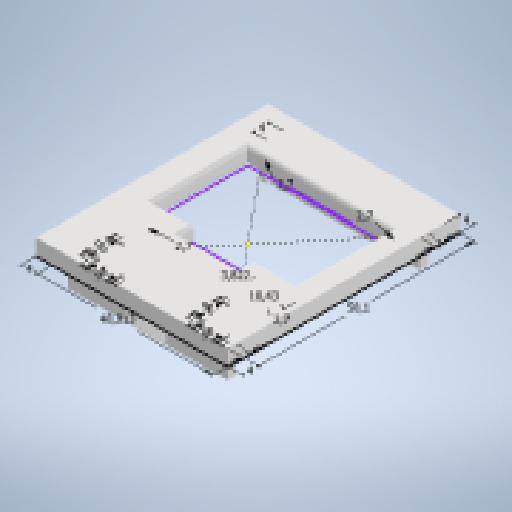
# Autodesk Inventor part: Deckel
Saved by Autodesk Inventor 2024 (Build 280153000, 153)
## iProperties
Created: 2025-05-07
Part Number: Deckel
Material: Generisch
Document SubType Name: Modeling
Designer: tobia
Density: 1 g/cm^3
Appearance: Vorgabe
Author: tobia
Autodesk Inventor part; units mm, degrees
ref_plane "YZ Plane" through (0, 0, 0) normal (1, 0, 0) x (0, 1, 0)
ref_plane "XZ Plane" through (0, 0, 0) normal (0, 1, 0) x (-1, 0, 0)
ref_plane "XY Plane" through (0, 0, 0) normal (0, 0, 1) x (1, 0, 0)
sketch "Skizze1" plane through (0, 0, 0) normal (0, 0, 1) x (1, 0, 0)
  line L0 (-24.0065, 29.05) -> (24.0065, 29.05)
  line L1 (24.0065, 29.05) -> (24.0065, -29.05)
  line L2 (24.0065, -29.05) -> (-24.0065, -29.05)
  line L3 (-24.0065, -29.05) -> (-24.0065, 29.05)
  line L4 (-24.0065, 29.05) -> (24.0065, -29.05) construction
  line L5 (24.0065, 29.05) -> (-24.0065, -29.05) construction
  line L6 (-24.0065, 29.05) -> (-20.0065, 29.05)
  line L7 (-20.0065, 29.05) -> (-20.0065, -29.05)
  line L8 (-20.0065, -29.05) -> (-24.0065, -29.05)
  line L9 (-24.0065, -29.05) -> (-24.0065, 29.05)
  line L10 (-20.0065, -29.05) -> (24.0065, -29.05)
  line L11 (24.0065, -29.05) -> (24.0065, -25.05)
  line L12 (24.0065, -25.05) -> (-20.0065, -25.05)
  line L13 (-20.0065, -25.05) -> (-20.0065, -29.05)
  line L14 (24.0065, -25.05) -> (20.0065, -25.05)
  line L15 (20.0065, -25.05) -> (20.0065, 29.05)
  line L16 (20.0065, 29.05) -> (24.0065, 29.05)
  line L17 (24.0065, 29.05) -> (24.0065, -25.05)
  line L18 (20.0065, 29.05) -> (-20.0065, 29.05)
  line L19 (-20.0065, 29.05) -> (-20.0065, 25.05)
  line L20 (-20.0065, 25.05) -> (20.0065, 25.05)
  line L21 (20.0065, 25.05) -> (20.0065, 29.05)
  line L22 (-20.0065, 25.05) -> (20.0065, 25.05)
  line L23 (20.0065, 25.05) -> (20.0065, 23.05)
  line L24 (20.0065, 23.05) -> (-20.0065, 23.05)
  line L25 (-20.0065, 23.05) -> (-20.0065, 25.05)
  line L26 (-20.0065, -25.05) -> (20.0065, -25.05)
  line L27 (20.0065, -25.05) -> (20.0065, -23.05)
  line L28 (20.0065, -23.05) -> (-20.0065, -23.05)
  line L29 (-20.0065, -23.05) -> (-20.0065, -25.05)
  line L30 (-24.0065, 29.05) -> (24.0065, 29.05)
  line L31 (24.0065, 29.05) -> (24.0065, -29.05)
  line L32 (24.0065, -29.05) -> (-24.0065, -29.05)
  line L33 (-24.0065, -29.05) -> (-24.0065, 29.05)
  circle A0 centre (-14.7085, 19.65) radius 1.35
  circle A1 centre (15.6927, 19.65) radius 1.35
  circle A2 centre (-14.7085, -8.9604) radius 1.35
  circle A3 centre (15.6927, -8.9604) radius 1.35
  line L34 (-17.3399, 17.2285) -> (18.4839, 17.2285)
  line L35 (18.4839, 17.2285) -> (18.4839, -6.4884)
  line L36 (18.4839, -6.4884) -> (-17.3399, -6.4884)
  line L37 (-17.3399, -6.4884) -> (-17.3399, 17.2285)
  line L38 (-17.3399, -6.4884) -> (-6.9094, -6.4884)
  line L39 (-6.9094, -10.3104) -> (-6.9094, -6.4884)
  line L40 (18.4839, -6.4884) -> (8.0539, -6.4884)
  line L41 (8.0539, -6.4884) -> (8.0539, -10.3104)
  line L42 (8.0539, -10.3104) -> (-6.9094, -10.3104)
  line L43 (-6.9094, 22.1958) -> (8.0539, 22.1958)
  line L44 (8.0539, 22.1958) -> (8.0539, 17.8498)
  line L45 (8.0539, 17.8498) -> (-6.9094, 17.8498)
  line L46 (-6.9094, 17.8498) -> (-6.9094, 22.1958)
  point P0 (0, 0)
  point P1 (-20.0065, -25.05)
  dimension "d0" = 48.013
  dimension "d1" = 58.1
  dimension "d2" = 4
  dimension "d3" = 4
  dimension "d4" = 4
  dimension "d5" = 4
  dimension "d6" = 2
  dimension "d7" = 2
  dimension "d28" = 2.7
  dimension "d29" = 2.7
  dimension "d30" = 2.7
  dimension "d31" = 2.7
  dimension "d32" = 10.43
  dimension "d33" = 3.822
  constraints: 94 end point, 20 parallel, 13 perpendicular, 10 horizontal, 8 point on line, 4 centre point, 2 midpoint
  measures "d0" distance of L1.end L2.end
  measures "d1" distance of L0.end L1.end
  measures "d2" distance of L7.end L8.end
  measures "d3" distance of L11.end L10.end
  measures "d4" distance of L15.end L16.end
  measures "d5" distance of L19.end L18.end
  measures "d6" distance of L22.end L23.end
  measures "d7" distance of L27.end L26.end
  measures "d28" diameter of A0
  measures "d29" diameter of A1
  measures "d30" diameter of A2
  measures "d31" diameter of A3
  measures "d32" distance of L35.end L40.end
  measures "d33" distance of L40.end L41.end
extrude "Extrusion1" add sketch "Skizze1" against normal blind 7 contours L20 L15 L24 L7 | L7 L28 L15 L12
sketch "Skizze2" plane through (-20.0065, -25.05, 0) normal (0, -1, 0) x (1, 0, 0)
  line L0 (40.013, 0) -> (0, 0) projected
  line L1 (40.013, 0) -> (20.013, 0)
  line L2 (20.013, 0) -> (20.013, -5)
  line L3 (15.513, -3.2) -> (24.513, -3.2)
  line L4 (24.513, -3.2) -> (24.513, -6.8)
  line L5 (24.513, -6.8) -> (15.513, -6.8)
  line L6 (15.513, -6.8) -> (15.513, -3.2)
  line L7 (15.513, -3.2) -> (24.513, -6.8) construction
  line L8 (24.513, -3.2) -> (15.513, -6.8) construction
  line L9 (20.013, -5) -> (15.513, -5)
  line L10 (20.013, -5) -> (24.513, -5)
  point P0 (20.0065, 0)
  dimension "d10" = 20
  dimension "d11" = 5
  dimension "d12" = 9
  dimension "d13" = 3.6
  constraints: 20 end point, 4 midpoint, 2 parallel, 2 perpendicular, 1 horizontal, 1 point on line
  measures "d10" distance of L0.start L1.end
  measures "d11" distance of L1.end L2.end
  measures "d12" distance of L4.end L5.end
  measures "d13" distance of L3.end L4.end
extrude "Extrusion2" add sketch "Skizze2" along normal blind 1.8
chamfer "Fasen1" distance 1.8 angle 45 2 edges at (0.0065, -26.85, -3.2) (0.0065, -26.85, -6.8)
sketch "Skizze3" plane through (-20.0065, 25.05, 0) normal (0, 1, 0) x (1, 0, 0)
  line L0 (40.013, 0) -> (40.013, 7) projected
  line L1 (40.013, 0) -> (20.013, 0)
  line L2 (0, 0) -> (40.013, 0) projected
  line L3 (20.013, 0) -> (20.013, 5)
  line L4 (24.513, 3.2) -> (15.513, 3.2)
  line L5 (15.513, 3.2) -> (15.513, 6.8)
  line L6 (15.513, 6.8) -> (24.513, 6.8)
  line L7 (24.513, 6.8) -> (24.513, 3.2)
  line L8 (24.513, 3.2) -> (15.513, 6.8) construction
  line L9 (15.513, 3.2) -> (24.513, 6.8) construction
  line L10 (20.013, 5) -> (24.513, 5)
  line L11 (24.513, 5) -> (15.513, 5)
  line L12 (15.513, 5) -> (15.513, 6.8)
  line L13 (15.513, 6.8) -> (24.513, 6.8)
  line L14 (24.513, 6.8) -> (24.513, 5)
  point P0 (20.0065, 0)
  dimension "d19" = 20
  dimension "d20" = 5
  dimension "d21" = 9
  dimension "d22" = 3.6
  constraints: 26 end point, 4 parallel, 3 midpoint, 3 perpendicular, 2 horizontal, 1 point on line
  measures "d19" distance of L0.start L1.end
  measures "d20" distance of L1.end L3.end
  measures "d21" distance of L5.end L6.end
  measures "d22" distance of L4.end L5.end
extrude "Extrusion3" add sketch "Skizze3" along normal blind 1.8
chamfer "Fasen2" distance 1.8 angle 45 2 edges at (0.0065, 26.85, -3.2) (0.0065, 26.85, -6.8)
extrude "Extrusion4" add sketch "Skizze1" along normal blind 4 contours L0 L7 L2 L3 | L0 L15 L20 L7 | L0 L1 L12 L15 | L20 L15 L24 L7 | L7 L12 L1 L2 | L24 L15 L28 L7 | L7 L28 L15 L12 | A0 | A1 | A2 | A3 | L34 L35 L36 L37 | L36 L41 L42 L39 | L43 L44 L45 L46
extrude "Extrusion5" add sketch "Skizze1" against normal blind 3 contours A0 | A1 | A2 | A3
extrude "Extrusion6" cut sketch "Skizze1" along normal blind 4 contours L34 L35 L36 L37 | L36 L41 L42 L39
fillet "Rundung1" radius 1 16 edges at (0.572, 17.2285, 4) (-17.3399, 5.3701, 4) (-12.1246, -6.4884, 4) (-6.9094, -8.3994, 4) (0.5723, -10.3104, 4) (8.0539, -8.3994, 4) (13.2689, -6.4884, 4) (18.4839, 5.3701, 4) (8.0539, -8.3994, 0) (13.2689, -6.4884, 0) (18.4839, 5.3701, 0) (0.5723, -10.3104, 0) (-12.1246, -6.4884, 0) (-6.9094, -8.3994, 0) (-17.3399, 5.3701, 0) (0.572, 17.2285, 0)
extrude "Extrusion7" cut sketch "Skizze1" along normal blind 3 contours L43 L44 L45 L46
sketch "Skizze4" plane through (0, 0, 0) normal (0, 0, -1) x (-1, 0, 0)
  line L0 (-17.7346, -15.3743) -> (-10.7346, -15.3743)
  line L1 (-10.7346, -15.3743) -> (-10.7346, -22.3743)
  line L2 (-10.7346, -22.3743) -> (-17.7346, -22.3743)
  line L3 (-17.7346, -22.3743) -> (-17.7346, -15.3743)
  line L4 (-17.7346, -15.3743) -> (-10.7346, -22.3743) construction
  line L5 (-10.7346, -15.3743) -> (-17.7346, -22.3743) construction
  line L6 (-18.7346, -14.3743) -> (-9.7346, -14.3743)
  line L7 (-9.7346, -14.3743) -> (-9.7346, -23.3743)
  line L8 (-9.7346, -23.3743) -> (-18.7346, -23.3743)
  line L9 (-18.7346, -23.3743) -> (-18.7346, -14.3743)
  line L10 (-18.7346, -14.3743) -> (-9.7346, -23.3743) construction
  line L11 (-9.7346, -14.3743) -> (-18.7346, -23.3743) construction
  line L12 (-17.2346, -15.8743) -> (-11.2346, -15.8743)
  line L13 (-11.2346, -15.8743) -> (-11.2346, -21.8743)
  line L14 (-11.2346, -21.8743) -> (-17.2346, -21.8743)
  line L15 (-17.2346, -21.8743) -> (-17.2346, -15.8743)
  line L16 (-17.2346, -15.8743) -> (-11.2346, -21.8743) construction
  line L17 (-11.2346, -15.8743) -> (-17.2346, -21.8743) construction
  line L18 (9.178, -15.8743) -> (15.178, -15.8743)
  line L19 (15.178, -15.8743) -> (15.178, -21.8743)
  line L20 (15.178, -21.8743) -> (9.178, -21.8743)
  line L21 (9.178, -21.8743) -> (9.178, -15.8743)
  line L22 (9.178, -15.8743) -> (15.178, -21.8743) construction
  line L23 (15.178, -15.8743) -> (9.178, -21.8743) construction
  line L24 (8.678, -15.3743) -> (15.678, -15.3743)
  line L25 (15.678, -15.3743) -> (15.678, -22.3743)
  line L26 (15.678, -22.3743) -> (8.678, -22.3743)
  line L27 (8.678, -22.3743) -> (8.678, -15.3743)
  line L28 (8.678, -15.3743) -> (15.678, -22.3743) construction
  line L29 (15.678, -15.3743) -> (8.678, -22.3743) construction
  line L30 (7.678, -14.3743) -> (16.678, -14.3743)
  line L31 (16.678, -14.3743) -> (16.678, -23.3743)
  line L32 (16.678, -23.3743) -> (7.678, -23.3743)
  line L33 (7.678, -23.3743) -> (7.678, -14.3743)
  line L34 (7.678, -14.3743) -> (16.678, -23.3743) construction
  line L35 (16.678, -14.3743) -> (7.678, -23.3743) construction
  point P0 (0, 0)
  point P1 (-14.2346, -18.8743)
  point P2 (-14.2346, -18.8743)
  point P3 (-14.2346, -18.8743)
  point P4 (12.178, -18.8743)
  point P5 (12.178, -18.8743)
  point P6 (12.178, -18.8743)
  dimension "d43" = 7
  dimension "d44" = 7
  dimension "d45" = 9
  dimension "d46" = 9
  dimension "d47" = 6
  dimension "d48" = 6
  dimension "d49" = 6
  dimension "d50" = 6
  dimension "d51" = 7
  dimension "d52" = 7
  dimension "d53" = 9
  dimension "d54" = 9
  constraints: 72 end point, 16 midpoint, 12 parallel, 6 horizontal, 6 perpendicular
  measures "d43" distance of L1.end L2.end
  measures "d44" distance of L0.end L1.end
  measures "d45" distance of L7.end L8.end
  measures "d46" distance of L6.end L7.end
  measures "d47" distance of L13.end L14.end
  measures "d48" distance of L12.end L13.end
  measures "d49" distance of L19.end L20.end
  measures "d50" distance of L18.end L19.end
  measures "d51" distance of L25.end L26.end
  measures "d52" distance of L24.end L25.end
  measures "d53" distance of L31.end L32.end
  measures "d54" distance of L30.end L31.end
extrude "Extrusion8" add sketch "Skizze4" along normal blind 5 contours L6 L7 L8 L9 | L30 L31 L32 L33
extrude "Extrusion9" add sketch "Skizze4" along normal blind 2 contours L0 L1 L2 L3 | L24 L25 L26 L27
extrude "Extrusion10" cut sketch "Skizze4" against normal blind 5 contours L12 L13 L14 L15 | L18 L19 L20 L21
fillet "Rundung2" radius 1 12 edges at (-12.178, -15.8743, 4) (-9.178, -18.8743, 4) (-12.178, -21.8743, 4) (-15.178, -18.8743, 4) (11.2346, -18.8743, 4) (14.2346, -15.8743, 4) (17.2346, -18.8743, 4) (14.2346, -21.8743, 4) (-24.0065, 0, 4) (0, -29.05, 4) (24.0065, 0, 4) (0, 29.05, 4)
